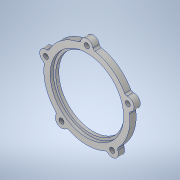
# Autodesk Inventor part: 조인트4베어링관절3
Saved by Autodesk Inventor 2020 (Build 240168000, 168)
## iProperties
Created: 2021-07-16
Part Number: 조인트4베어링관절3
Material: 알루미늄 6061
Document SubType Name: Modeling
Designer: user
Density: 2.7 g/cm^3
Appearance: 알루미늄 - 평지
Mass: 9.02885 g
Surface Area: 34.5411 cm^2
Volume: 3.34402 cm^3
Author: user
Autodesk Inventor part; units mm, degrees
ref_plane "YZ Plane" through (0, 0, 0) normal (1, 0, 0) x (0, 1, 0)
ref_plane "XZ Plane" through (0, 0, 0) normal (0, 1, 0) x (-1, 0, 0)
ref_plane "XY Plane" through (0, 0, 0) normal (0, 0, 1) x (1, 0, 0)
sketch "스케치1" plane through (0, 0, 0) normal (0, 0, 1) x (1, 0, 0)
  circle A0 centre (0, 0) radius 22
  circle A1 centre (0, 0) radius 23.525
  circle A2 centre (0, 0) radius 27.6
  line L0 (0, 0) -> (0, 27.6)
  circle A3 centre (0, 27.6) radius 1.25
  circle A4 centre (0, 27.6) radius 4
  circle A5 centre (-26.2492, 8.5289) radius 4
  circle A6 centre (-26.2492, 8.5289) radius 1.25
  circle A7 centre (-16.2229, -22.3289) radius 4
  circle A8 centre (-16.2229, -22.3289) radius 1.25
  circle A9 centre (16.2229, -22.3289) radius 4
  circle A10 centre (16.2229, -22.3289) radius 1.25
  circle A11 centre (26.2492, 8.5289) radius 4
  circle A12 centre (26.2492, 8.5289) radius 1.25
  dimension "d2" = 55.2
  dimension "d0" = 44
  dimension "d1" = 47.05
  dimension "d3" = 2.5
  dimension "d4" = 8
  dimension "d7" = 360
  constraints: 12 centre point, 9 coincident, 2 end point, 1 vertical, 1 vertical alignment, 23 other
  measures "d0" diameter of A0
  measures "d1" diameter of A1
  measures "d3" diameter of A3
  measures "d4" diameter of A4
extrude "돌출1" add sketch "스케치1" along normal blind 2 contours A1 | A2 A9 A7 A5 A4 A11 | A11 A2 A12 | A2 A12 A11 | A9 A2 A10 | A2 A10 A9 | A12 A2 | A2 A12 | A10 A2 | A2 A10 | A4 L0 A3 A2 | A2 A3 A4 | A7 A2 A8 | A2 A8 A7 | A3 L0 A2 | A2 A3 | A4 A2 A3 L0 | A8 A2 | A2 A8 | L0 A3 A2 | A5 A2 A6 | A2 A6 A5 | A6 A2 | A2 A6
sketch "스케치2" plane through (0, 0, 2) normal (0, 0, 1) x (1, 0, 0)
  circle A0 centre (0, 0) radius 23.535
  circle A1 centre (0, 0) radius 27.6
  circle A2 centre (0, 0) radius 22 projected
  arc A3 (19.2801, -19.7494) -> (27.2063, 4.6451) centre (0, 0) ccw projected
  arc A4 (27.2063, 4.6451) -> (24.7407, 12.2335) centre (26.2492, 8.5289) ccw projected
  arc A5 (24.7407, 12.2335) -> (3.9895, 27.3101) centre (0, 0) ccw projected
  arc A6 (3.9895, 27.3101) -> (-3.9895, 27.3101) centre (0, 27.6) ccw projected
  arc A7 (-3.9895, 27.3101) -> (-24.7407, 12.2335) centre (0, 0) ccw projected
  arc A8 (-24.7407, 12.2335) -> (-27.2063, 4.6451) centre (-26.2492, 8.5289) ccw projected
  arc A9 (-27.2063, 4.6451) -> (-19.2801, -19.7494) centre (0, 0) ccw projected
  arc A10 (-19.2801, -19.7494) -> (-12.8249, -24.4393) centre (-16.2229, -22.3289) ccw projected
  arc A11 (-12.8249, -24.4393) -> (12.8249, -24.4393) centre (0, 0) ccw projected
  arc A12 (12.8249, -24.4393) -> (19.2801, -19.7494) centre (16.2229, -22.3289) ccw projected
  circle A13 centre (0, 27.6) radius 4
  circle A14 centre (26.2492, 8.5289) radius 4
  circle A15 centre (-26.2492, 8.5289) radius 4
  circle A16 centre (-16.2229, -22.3289) radius 4
  circle A17 centre (16.2229, -22.3289) radius 4
  dimension "d11" = 47.07
  dimension "d12" = 55.2
  dimension "d13" = 8
  dimension "d14" = 8
  dimension "d15" = 8
  dimension "d16" = 8
  dimension "d17" = 8
  constraints: 7 centre point, 7 coincident
  measures "d11" diameter of A0
  measures "d12" diameter of A1
  measures "d13" diameter of A13
  measures "d14" diameter of A14
  measures "d15" diameter of A15
  measures "d16" diameter of A16
  measures "d17" diameter of A17
extrude "돌출2" add sketch "스케치2" along normal blind 2 contours A1 A17 A16 A15 A13 A14 | A14 A1 | A1 A4 | A12 A1 | A1 A17 | A13 A1 | A1 A6 | A10 A1 | A1 A16 | A15 A1 | A1 A8
sketch "스케치3" plane through (0, 0, 4) normal (0, 0, 1) x (1, 0, 0)
  circle A0 centre (0, 0) radius 23.535 projected
  arc A1 (24.7407, 12.2335) -> (3.9895, 27.3101) centre (0, 0) ccw projected
  arc A2 (3.9895, 27.3101) -> (-3.9895, 27.3101) centre (0, 27.6) ccw projected
  arc A3 (-3.9895, 27.3101) -> (-24.7407, 12.2335) centre (0, 0) ccw projected
  arc A4 (-24.7407, 12.2335) -> (-27.2063, 4.6451) centre (-26.2492, 8.5289) ccw projected
  arc A5 (-27.2063, 4.6451) -> (-19.2801, -19.7494) centre (0, 0) ccw projected
  arc A6 (-19.2801, -19.7494) -> (-12.8249, -24.4393) centre (-16.2229, -22.3289) ccw projected
  arc A7 (-12.8249, -24.4393) -> (12.8249, -24.4393) centre (0, 0) ccw projected
  arc A8 (12.8249, -24.4393) -> (19.2801, -19.7494) centre (16.2229, -22.3289) ccw projected
  arc A9 (19.2801, -19.7494) -> (27.2063, 4.6451) centre (0, 0) ccw projected
  arc A10 (27.2063, 4.6451) -> (24.7407, 12.2335) centre (26.2492, 8.5289) ccw projected
  circle A11 centre (-26.2492, 8.5289) radius 1.6
  circle A12 centre (0, 27.6) radius 1.6
  circle A13 centre (26.2492, 8.5289) radius 1.6
  circle A14 centre (16.2229, -22.3289) radius 1.6
  circle A15 centre (-16.2229, -22.3289) radius 1.6
  dimension "d20" = 3.2
  dimension "d21" = 3.2
  dimension "d22" = 3.2
  dimension "d23" = 3.2
  dimension "d24" = 3.2
  constraints: 5 centre point, 5 coincident
  measures "d20" diameter of A11
  measures "d21" diameter of A12
  measures "d22" diameter of A13
  measures "d23" diameter of A14
  measures "d24" diameter of A15
extrude "돌출3" cut sketch "스케치3" against normal up to surface (4 mm away) contours A11 | A12 | A13 | A14 | A15
fillet "모깎기1" radius 1.5 10 edges at (24.7407, 12.2335, 2) (27.2063, 4.6451, 2) (3.9895, 27.3101, 2) (-3.9895, 27.3101, 2) (-24.7407, 12.2335, 2) (-27.2063, 4.6451, 2) (-19.2801, -19.7494, 2) (-12.8249, -24.4393, 2) (19.2801, -19.7494, 2) (12.8249, -24.4393, 2)
chamfer "모따기1" distance 1.5 angle 45 5 edges at (-27.8492, 8.5289, 0) (-1.6, 27.6, 0) (24.6492, 8.5289, 0) (14.6229, -22.3289, 0) (-17.8229, -22.3289, 0)
